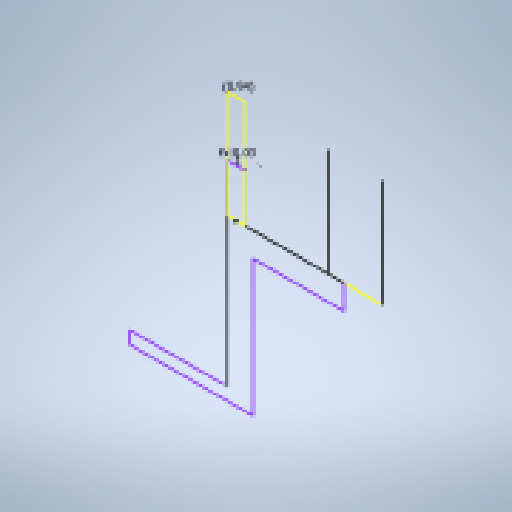
# Autodesk Inventor part: j1 enndstop blocker
Saved by Autodesk Inventor 2025 (Build 290162000, 162)
## iProperties
Created: 2025-07-09
Part Number: j1 enndstop blocker
Material: 一般
Document SubType Name: Modeling
Designer: gavin
Density: 1 g/cm^3
Appearance: 預設
Author: gavin
Autodesk Inventor part; units mm, degrees
ref_plane "YZ Plane" through (0, 0, 0) normal (1, 0, 0) x (0, 1, 0)
ref_plane "XZ Plane" through (0, 0, 0) normal (0, 1, 0) x (-1, 0, 0)
ref_plane "XY Plane" through (0, 0, 0) normal (0, 0, 1) x (1, 0, 0)
sketch "草圖1" plane through (0, 0, 0) normal (0, 0, 1) x (1, 0, 0)
  line L0 (-0.3223, -18.9936) -> (-5.7251, -18.9936)
  line L1 (-5.7251, -18.9936) -> (-5.7251, -20.1936)
  line L2 (-5.7251, -20.1936) -> (1.1777, -20.1936)
  line L3 (1.1777, -20.1936) -> (1.1777, -7.3911)
  line L4 (1.1777, -7.3911) -> (8.6477, -7.3911)
  line L5 (8.6477, -7.3911) -> (8.6477, -5.8911)
  line L6 (8.6477, -5.8911) -> (0.6777, -5.9936)
  line L7 (0.6777, -5.9936) -> (0.6777, -2.9936)
  line L8 (0.6777, -2.9936) -> (-0.3223, -2.9936)
  line L9 (-0.3223, -2.9936) -> (-0.3223, -18.9936)
  line L10 (0.6477, -6) -> (-0.2923, -6) projected
  line L11 (0.6477, 0) -> (0.6477, -6) projected
  line L12 (-0.2923, 0) -> (0.6477, 0) projected
  line L13 (-0.2923, 0) -> (-0.2923, -6) projected
  line L14 (4.1477, 0) -> (7.1477, 0) projected
  line L15 (4.1477, 0) -> (4.1477, -6)
  line L16 (7.1477, 0) -> (7.1477, -6)
  line L17 (7.1477, -6) -> (4.1477, -6) projected
  point P0 (0.1784, -6)
  point P1 (0.1777, -6)
  point P2 (8.6477, -6.6411)
  dimension "d0" = 1
  dimension "d3" = 0.94
  dimension "d4" = 0.03
  dimension "d5" = 3
  dimension "d6" = 1.5
  dimension "d7" = 1.2
  dimension "d8" = 16
  dimension "d9" = 1.5
  dimension "d10" = 1.5
  constraints: 22 end point, 5 perpendicular, 3 vertical, 2 midpoint, 1 horizontal, 1 parallel, 8 other
  measures "d0" distance of L7.end L8.end
  measures "d3" distance of L12.start L11.start
  measures "d4" distance between parallel lines of L7 L11
  measures "d5" distance of L7.start L7.end
  measures "d6" distance from line of L16 point (8.648, -6.641)
  measures "d7" distance of L0.end L1.end
  measures "d8" distance of L8.end L0.start
  measures "d9" distance of L4.end L5.end
  measures "d10" distance between parallel lines of L3 L9
extrude "擠出1" add sketch "草圖1" along normal blind 6 contours L9 L8 L13 L10 L11 L7 L6 L15 L17 L16 L5 L4 L3 L2 L1 L0 | L8 L11 L10 L13 | L6 L16 L17 L15
fillet "圓角1" radius 3 2 edges at (8.6477, -6.6411, 6) (8.6477, -6.6411, 0)
sketch "草圖3" plane through (0.6777, -5.9936, 6) normal (-0.0128564, 0.9999174, 0) x (0.9999174, 0.0128564, 0)
  ellipse E0 centre (5.0466, 3) end of major axis (5.0466, 1.5) minor radius 1.4999 construction
  ellipse E1 centre (4.9695, 3) end of major axis (4.9695, 4.5) minor radius 1.4999 projected
  point P0 (-0.6006, 6)
  constraints: 1 other
extrude "擠出2" cut sketch "草圖3" against normal up to surface (1.4326 mm away)
equation "\"d4\" = -0.5 * d3 + 0.5 * d0"
